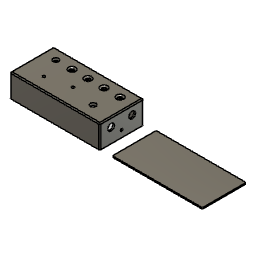
Echobase case v1 (Autodesk Fusion 360 design; units mm, degrees)
Autodesk Fusion 360 part; units mm, degrees
sketch "Sketch3" plane through (0, 0, 0) normal (0, 1, 0) x (1, 0, 0)
  line L0 (-86.0512, 43.1396) -> (88.9488, 43.1396)
  line L1 (88.9488, 43.1396) -> (88.9488, -41.8604)
  line L2 (88.9488, -41.8604) -> (-86.0512, -41.8604)
  line L3 (-86.0512, -41.8604) -> (-86.0512, 43.1396)
  dimension "d7" = 175
  dimension "d8" = 85
  constraint horizontal L0
  constraint vertical L1
  constraint horizontal L2
  constraint vertical L3
  measures "d7" distance of L0.start L0.end
  measures "d8" distance of L0.start L2.end
extrude "Extrude2" add sketch "Sketch3" along normal blind 45 makes body 1
sketch "Sketch4" plane through (0, 0, 0) normal (0, -1, 0) x (1, 0, 0)
  line L0 (88.9488, 41.8604) -> (-86.0512, 41.8604)
  line L1 (-86.0512, 41.8604) -> (-86.0512, -43.1396)
  line L2 (-86.0512, -43.1396) -> (88.9488, -43.1396)
  line L3 (88.9488, -43.1396) -> (88.9488, 41.8604)
  line L4 (-83.0512, 38.8604) -> (85.9488, 38.8604)
  line L5 (85.9488, 38.8604) -> (85.9488, -40.1396)
  line L6 (85.9488, -40.1396) -> (-83.0512, -40.1396)
  line L7 (-83.0512, -40.1396) -> (-83.0512, 38.8604)
  dimension "d11" = 169
  dimension "d12" = 79
  dimension "d13" = 3
  dimension "d14" = 3
  constraint horizontal L4
  constraint vertical L5
  constraint horizontal L6
  constraint vertical L7
  measures "d11" distance of L4.start L4.end
  measures "d12" distance of L4.start L6.end
  measures "d13" distance of L1 L7
  measures "d14" distance of L2 L6
extrude "Extrude3" cut sketch "Sketch4" against normal blind 40 contours L4 L5 L6 L7 bodies 1
sketch "Sketch5" plane through (0, 45, 0) normal (0, 1, 0) x (-1, 0, 0)
  line L0 (86.0512, 41.8604) -> (-88.9488, 41.8604)
  line L1 (-88.9488, 41.8604) -> (-88.9488, -43.1396)
  line L2 (-88.9488, -43.1396) -> (86.0512, -43.1396)
  line L3 (86.0512, -43.1396) -> (86.0512, 41.8604)
  circle A0 centre (61.0512, -22.6716) radius 5.5
  circle A1 centre (29.8012, -22.6386) radius 3.5
  circle A2 centre (-1.4488, -22.5681) radius 3.5
  circle A3 centre (-32.6988, -22.5514) radius 3.5
  circle A4 centre (-63.9488, -22.4643) radius 3.5
  circle A5 centre (29.8012, -22.6386) radius 7
  circle A6 centre (-1.4488, -22.5681) radius 7
  circle A7 centre (-32.6988, -22.5514) radius 7
  circle A8 centre (-63.9488, -22.4643) radius 7
  dimension "d17" = 11
  dimension "d19" = 7
  dimension "d20" = 7
  dimension "d21" = 7
  dimension "d22" = 7
  dimension "d23" = 25
  dimension "d24" = 25
  dimension "d25" = 31.25
  dimension "d26" = 31.25
  dimension "d27" = 31.25
  dimension "d30" = 14
  dimension "d31" = 14
  dimension "d32" = 14
  dimension "d33" = 14
  constraint concentric A1 A5
  constraint concentric A2 A6
  constraint concentric A3 A7
  constraint concentric A4 A8
  measures "d17" diameter of A0
  measures "d19" diameter of A1
  measures "d20" diameter of A2
  measures "d21" diameter of A3
  measures "d22" diameter of A4
  measures "d23" distance of L1 A4.centre
  measures "d24" distance of L3 A0.centre
  measures "d25" horizontal distance of A0.centre A1.centre
  measures "d26" horizontal distance of A1.centre A2.centre
  measures "d27" horizontal distance of A2.centre A3.centre
  measures "d30" diameter of A5
  measures "d31" diameter of A6
  measures "d32" diameter of A7
  measures "d33" diameter of A8
extrude "Extrude4" cut sketch "Sketch5" against normal blind 5 contours A0 | A1 | A2 | A3 | A4 bodies 1
extrude "Extrude5" cut sketch "Sketch5" against normal blind 2.5 contours A5 | A6 | A7 | A8 bodies 1
chamfer "Chamfer1" distance 2.5 angle 45 1 edges at (-23.2749, 42.5, -20.1072) on bodies 1
chamfer "Chamfer2" distance 2.5 angle 45 1 edges at (7.9751, 42.5, -20.0368) on bodies 1
chamfer "Chamfer3" distance 2.5 angle 45 1 edges at (39.2251, 42.5, -20.0201) on bodies 1
chamfer "Chamfer4" distance 2.5 angle 45 1 edges at (70.4751, 42.5, -19.933) on bodies 1
sketch "Sketch6" plane through (0, 45, 0) normal (0, 1, 0) x (-1, 0, 0)
  circle A0 centre (-1.4488, -22.5681) radius 7
  circle A1 centre (-32.6988, -22.5514) radius 7
  circle A2 centre (29.8012, -22.6386) radius 7
  circle A3 centre (-63.9488, -22.4643) radius 7
  circle A4 centre (61.0512, -22.6716) radius 5.5
  line L0 (86.0512, 41.8604) -> (-88.9488, 41.8604)
  line L1 (-88.9488, 41.8604) -> (-88.9488, -43.1396)
  line L2 (-88.9488, -43.1396) -> (86.0512, -43.1396)
  line L3 (86.0512, -43.1396) -> (86.0512, 41.8604)
  circle A5 centre (-1.4518, 6.801) radius 2.5
  dimension "d41" = 5
  measures "d41" diameter of A5
extrude "Extrude6" cut sketch "Sketch6" against normal blind 5 contours A5 bodies 1
sketch "Sketch7" plane through (0, 45, 0) normal (0, 1, 0) x (-1, 0, 0)
  circle A0 centre (-1.4518, 6.801) radius 2.5
  circle A1 centre (-1.4488, -22.5681) radius 7
  circle A2 centre (-32.6988, -22.5514) radius 7
  circle A3 centre (29.8012, -22.6386) radius 7
  circle A4 centre (-63.9488, -22.4643) radius 7
  circle A5 centre (61.0512, -22.6716) radius 5.5
  line L0 (86.0512, 41.8604) -> (-88.9488, 41.8604)
  line L1 (-88.9488, 41.8604) -> (-88.9488, -43.1396)
  line L2 (-88.9488, -43.1396) -> (86.0512, -43.1396)
  line L3 (86.0512, -43.1396) -> (86.0512, 41.8604)
  circle A6 centre (45.0026, 16.8265) radius 2.5
  dimension "d44" = 5
  measures "d44" diameter of A6
extrude "Extrude7" cut sketch "Sketch7" against normal blind 5 contours A6 bodies 1
sketch "Sketch8" plane through (0, 45, 0) normal (0, 1, 0) x (-1, 0, 0)
  circle A0 centre (45.0026, 16.8265) radius 2.5
  circle A1 centre (-1.4518, 6.801) radius 2.5
  circle A2 centre (-1.4488, -22.5681) radius 7
  circle A3 centre (-32.6988, -22.5514) radius 7
  circle A4 centre (29.8012, -22.6386) radius 7
  circle A5 centre (-63.9488, -22.4643) radius 7
  circle A6 centre (61.0512, -22.6716) radius 5.5
  line L0 (86.0512, 41.8604) -> (-88.9488, 41.8604)
  line L1 (-88.9488, 41.8604) -> (-88.9488, -43.1396)
  line L2 (-88.9488, -43.1396) -> (86.0512, -43.1396)
  line L3 (86.0512, -43.1396) -> (86.0512, 41.8604)
  circle A7 centre (-50.943, 16.7783) radius 5.5
  dimension "d47" = 11
  measures "d47" diameter of A7
extrude "Extrude8" cut sketch "Sketch8" against normal blind 5 contours A7 bodies 1
sketch "Sketch9" plane through (88.9488, 0, 0) normal (1, 0, 0) x (0, 0, -1)
  line L0 (-41.8604, 0) -> (43.1396, 0)
  line L1 (43.1396, 0) -> (43.1396, 45)
  line L2 (43.1396, 45) -> (-41.8604, 45)
  line L3 (-41.8604, 45) -> (-41.8604, 0)
  circle A0 centre (0.6396, 13) radius 2.5
  dimension "d50" = 5
  dimension "d51" = 42.5
  dimension "d52" = 13
  measures "d50" diameter of A0
  measures "d51" distance of L3 A0.centre
  measures "d52" distance of L0 A0.centre
extrude "Extrude9" cut sketch "Sketch9" against normal blind 3 contours A0 bodies 1
sketch "Sketch10" plane through (88.9488, 0, 0) normal (1, 0, 0) x (0, 0, -1)
  circle A0 centre (0.6396, 13) radius 2.5
  line L0 (-41.8604, 0) -> (43.1396, 0)
  line L1 (43.1396, 0) -> (43.1396, 45)
  line L2 (43.1396, 45) -> (-41.8604, 45)
  line L3 (-41.8604, 45) -> (-41.8604, 0)
  circle A1 centre (-19.8604, 28) radius 6.5
  circle A2 centre (21.1396, 28) radius 6.5
  dimension "d55" = 13
  dimension "d56" = 28
  dimension "d57" = 22
  dimension "d58" = 13
  dimension "d59" = 22
  dimension "d60" = 28
  measures "d55" diameter of A1
  measures "d56" distance of L0 A1.centre
  measures "d57" distance of L3 A1.centre
  measures "d58" diameter of A2
  measures "d59" distance of L1 A2.centre
  measures "d60" distance of L0 A2.centre
extrude "Extrude10" cut sketch "Sketch10" against normal blind 3 contours A1 | A2 bodies 1
fillet "Fillet1" radius 2 8 edges at (88.9488, 22.5, 41.8604) (88.9488, 45, -0.6396) (1.4488, 45, 41.8604) (88.9488, 22.5, -43.1396) (1.4488, 45, -43.1396) (-86.0512, 22.5, 41.8604) (-86.0512, 45, -0.6396) (-86.0512, 22.5, -43.1396) on bodies 1
sketch "Sketch11" plane through (0, 0, 0) normal (0, 1, 0) x (1, 0, 0)
  line L0 (113.5035, 43.1807) -> (288.5035, 43.1807)
  line L1 (288.5035, 43.1807) -> (288.5035, -41.8193)
  line L2 (288.5035, -41.8193) -> (113.5035, -41.8193)
  line L3 (113.5035, -41.8193) -> (113.5035, 43.1807)
  dimension "d65" = 175
  dimension "d66" = 85
  constraint horizontal L0
  constraint vertical L1
  constraint horizontal L2
  constraint vertical L3
  measures "d65" distance of L0.start L0.end
  measures "d66" distance of L0.start L2.end
extrude "Extrude11" add sketch "Sketch11" along normal blind 3 separate body makes body 2
fillet "Fillet2" radius 2 4 edges at (288.5035, 1.5, 41.8193) (288.5035, 1.5, -43.1807) (113.5035, 1.5, 41.8193) (113.5035, 1.5, -43.1807) on bodies 2
fillet "Fillet3" radius 0.5 8 edges at (287.9177, 0, -42.5949) (288.5035, 0, -0.6807) (287.9177, 0, 41.2336) (201.0035, 0, 41.8193) (114.0892, 0, 41.2336) (113.5035, 0, -0.6807) (114.0892, 0, -42.5949) (201.0035, 0, -43.1807) on bodies 2
